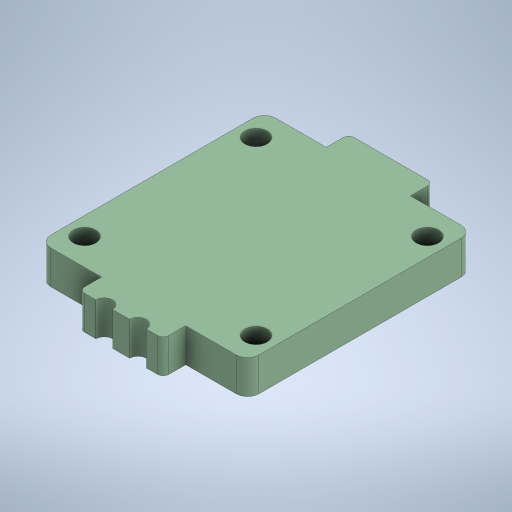
# Autodesk Inventor part: Holybro Tekko ESC model
Saved by Autodesk Inventor 2024 (Build 280153000, 153)
## iProperties
Created: 2024-03-12
Part Number: Holybro Tekko ESC model
Material: PMMA Plastic
Document SubType Name: Modeling
Designer: nicoe
Mass: 10.9655 g
Surface Area: 43.8799 cm^2
Volume: 9.23024 cm^3
Density: 1.188 g/cm^3
Appearance: Rubber - Green
Author: nicoe
Autodesk Inventor part; units mm, degrees
ref_plane "YZ Plane" through (0, 0, 0) normal (1, 0, 0) x (0, 1, 0)
ref_plane "XZ Plane" through (0, 0, 0) normal (0, 1, 0) x (-1, 0, 0)
ref_plane "XY Plane" through (0, 0, 0) normal (0, 0, 1) x (1, 0, 0)
sketch "Sketch1" plane through (0, 0, 0) normal (0, 1, 0) x (-1, 0, 0)
  line L0 (16.5, 20) -> (-16.5, 20)
  line L1 (-18.5, 18) -> (-18.5, -18)
  line L2 (-16.5, -20) -> (16.5, -20)
  line L3 (18.5, -18) -> (18.5, 18)
  arc A0 (18.5, 18) -> (16.5, 20) centre (16.5, 18) ccw
  arc A1 (16.5, -20) -> (18.5, -18) centre (16.5, -18) ccw
  arc A2 (-16.5, 20) -> (-18.5, 18) centre (-16.5, 18) ccw
  arc A3 (-18.5, -18) -> (-16.5, -20) centre (-16.5, -18) ccw
  line L4 (6.5, 24) -> (-6.5, 24)
  line L5 (-7.5, 23) -> (-7.5, 20)
  line L6 (-7.5, 20) -> (7.5, 20)
  line L7 (7.5, 20) -> (7.5, 23)
  line L8 (7.5, -20) -> (-7.5, -20)
  line L9 (-7.5, -20) -> (-7.5, -23)
  line L10 (-6.5, -24) -> (6.5, -24)
  line L11 (7.5, -23) -> (7.5, -20)
  arc A4 (7.5, 23) -> (6.5, 24) centre (6.5, 23) ccw
  arc A5 (-6.5, 24) -> (-7.5, 23) centre (-6.5, 23) ccw
  arc A6 (-7.5, -23) -> (-6.5, -24) centre (-6.5, -23) ccw
  arc A7 (6.5, -24) -> (7.5, -23) centre (6.5, -23) ccw
  circle A8 centre (3, 24) radius 1.5
  circle A9 centre (-3, 24) radius 1.5
  circle A10 centre (15.25, 15.25) radius 2
  circle A11 centre (15.25, -15.25) radius 2
  circle A12 centre (-15.25, -15.25) radius 2
  circle A13 centre (-15.25, 15.25) radius 2
  point P0 (0, 0)
  point P1 (-18.5, -20)
  point P2 (-18.5, 20)
  point P3 (18.5, -20)
  point P4 (-7.5, 24)
  point P5 (-7.5, -24)
  point P6 (7.5, -24)
  point P7 (0, 20)
  point P8 (0, -20)
  point P9 (4.5, 24)
  point P10 (1.5, 24)
  point P11 (-1.5, 24)
  point P12 (-4.5, 24)
  dimension "d0" = 37
  dimension "d1" = 40
  dimension "d2" = 20
  dimension "d3" = 18.5
  dimension "d4" = 2
  dimension "d5" = 15
  dimension "d6" = 4
  dimension "d7" = 15
  dimension "d8" = 4
  dimension "d9" = 1
  dimension "d10" = 3
  dimension "d11" = 3
  dimension "d12" = 3
  dimension "d13" = 6
  dimension "d14" = 4
  dimension "d15" = 4
  dimension "d16" = 4
  dimension "d17" = 4
  dimension "d18" = 30.5
  dimension "d19" = 30.5
  dimension "d20" = 30.5
  dimension "d21" = 30.5
  dimension "d22" = 3.25
  dimension "d23" = 4.75
  constraints: 24 end point, 16 point on circle, 16 tangent, 14 centre point, 14 point on line, 6 equal radius, 6 parallel, 4 midpoint, 3 horizontal, 3 perpendicular, 1 horizontal alignment, 1 vertical alignment
  measures "d0" distance of point (18.5, -20) point (-18.5, -20)
  measures "d1" distance of point (-18.5, -20) point (-18.5, 20)
  measures "d2" distance from line of L2 point (0, 0)
  measures "d3" distance from line of L3 point (0, 0)
  measures "d4" radius of A0
  measures "d5" distance of L6.end L5.end
  measures "d6" distance of L5.end point (-7.5, 24)
  measures "d7" distance of point (7.5, -24) point (-7.5, -24)
  measures "d8" distance of point (-7.5, -24) L8.end
  measures "d9" radius of A4
  measures "d10" diameter of A8
  measures "d11" diameter of A9
  measures "d12" horizontal distance of point (0, 0) A9.centre
  measures "d13" distance of A8.centre A9.centre
  measures "d14" diameter of A10
  measures "d15" diameter of A11
  measures "d16" diameter of A12
  measures "d17" diameter of A13
  measures "d18" distance of A11.centre A10.centre
  measures "d19" distance of A13.centre A12.centre
  measures "d20" distance of A11.centre A12.centre
  measures "d21" distance of A10.centre A13.centre
  measures "d22" distance from line of L3 A11.centre
  measures "d23" distance from line of L2 A11.centre
extrude "Extrusion1" add sketch "Sketch1" along normal blind 6 contours A0 L3 A1 L2 A3 L1 A2 L0 | L0 L5 A5 L4 A9 A8 A4 L7 | L11 A7 L10 A6 L9 L2
equation "\"d2\" = 0.5 * d1"
equation "\"d3\" = 0.5 * d0"
equation "\"d22\" = -0.5 * d20 + 0.5 * d0"
equation "\"d23\" = -0.5 * d19 + 0.5 * d1"
body "Solid1"
